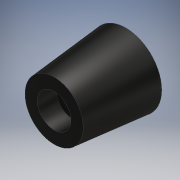
# Autodesk Inventor part: cleat
Saved by Autodesk Inventor 2018 (Build 220112000, 112)
## iProperties
Created: 2018-05-01
Part Number: cleat
Material: Generic
Document SubType Name: Modeling
Designer: medrimonia
Density: 1 g/cm^3
Appearance: Glossy - Black
Vendor: Rhoban
Mass: 2.72317 g
Surface Area: 14.1383 cm^2
Volume: 2.72317 cm^3
Author: medrimonia
Autodesk Inventor part; units mm, degrees
ref_plane "YZ Plane" through (0, 0, 0) normal (1, 0, 0) x (0, 1, 0)
ref_plane "XZ Plane" through (0, 0, 0) normal (0, 1, 0) x (-1, 0, 0)
ref_plane "XY Plane" through (0, 0, 0) normal (0, 0, 1) x (1, 0, 0)
sketch "Sketch1" plane through (0, 0, 0) normal (0, 0, 1) x (1, 0, 0)
  line L0 (6.5, 0) -> (-6.5, 0)
  line L1 (-6.5, 0) -> (-8, 16)
  line L2 (-8, 16) -> (8, 16)
  line L3 (8, 16) -> (6.5, 0)
  line L4 (0, 0) -> (0, 16)
  dimension "d1" = 13
  dimension "d2" = 16
  dimension "d3" = 16
  constraints: 10 end point, 2 midpoint, 1 coincident, 1 horizontal, 1 parallel, 1 vertical
  measures "d1" distance of L0.start L0.end
  measures "d2" distance of L1.end L2.end
  measures "d3" distance of L4.start L4.end
revolve "Revolution1" add sketch "Sketch1" angle 360 about axis through (0, 0, 0) along (0, 1, 0) contours L0 L1 L2 L4
sketch "Sketch2" plane through (0, 0, 0) normal (0, -1, 0) x (1, 0, 0)
  circle A0 centre (0, 0) radius 6.5 projected
hole "Hole1" at (0, 0, 0) direction (0, 1, 0) diameter 4.5 end through all counterbore diameter 7.5 counterbore depth 4.2
equation "\"d1\" = cleat_base_diameter"
equation "\"d2\" = cleat_top_diameter"
equation "\"d3\" = cleat_height"
equation "\"d5\" = hole_diameter"
equation "\"d7\" = trace_diameter"
equation "\"d8\" = trace_depth"
equation "\"hole_diameter\" = 4.5"
equation "\"cleat_height\" = 16"
equation "\"trace_diameter\" = 7.5"
equation "\"trace_depth\" = 4.2"
equation "\"cleat_base_diameter\" = 13"
equation "\"cleat_top_diameter\" = 16"
body "Solid1"
